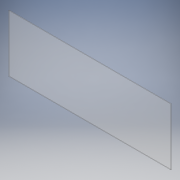
# Autodesk Inventor part: Front Panel Window
Saved by Autodesk Inventor 2018 (Build 220112000, 112)
## iProperties
Created: 2018-08-09
Part Number: Front Panel Window
Material: Polycarbonate, Clear
Document SubType Name: Modeling
Designer: P301319
Density: 1.2 g/cm^3
Appearance: Polycarbonate - Clear
Author: P301319
Autodesk Inventor part; units mm, degrees
ref_plane "YZ Plane" through (0, 0, 0) normal (1, 0, 0) x (0, 1, 0)
ref_plane "XZ Plane" through (0, 0, 0) normal (0, 1, 0) x (-1, 0, 0)
ref_plane "XY Plane" through (0, 0, 0) normal (0, 0, 1) x (1, 0, 0)
sketch "Sketch1" plane through (0, 0, 0) normal (0, 0, 1) x (1, 0, 0)
  line L0 (0, 0) -> (1080, 0)
  line L1 (1080, 0) -> (1080, 380)
  line L2 (1080, 380) -> (0, 380)
  line L3 (0, 380) -> (0, 0)
  dimension "d0" = 1080
  dimension "d1" = 380
  constraints: 8 end point, 2 parallel, 1 horizontal, 1 perpendicular
  measures "d0" distance of L2.end L1.end
  measures "d1" distance of L1.end L0.end
extrude "Extrusion1" add sketch "Sketch1" along normal blind 4
body "Solid1"
